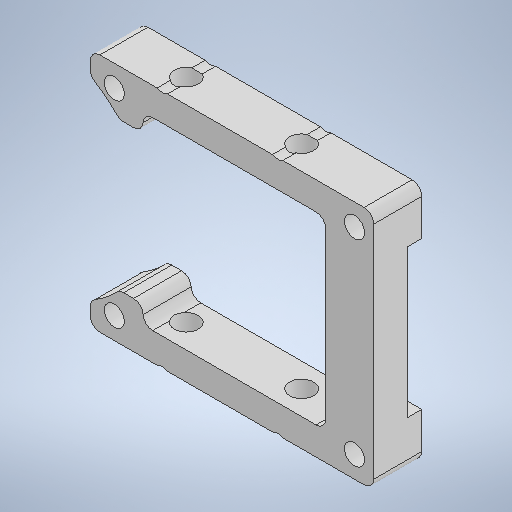
# Autodesk Inventor part: AP3.0_servo-mount
Saved by Autodesk Inventor 2025.1 (Build 291241020, 241B)
## iProperties
Created: 2024-04-22
Part Number: AP3.0_servo-mount
Material: 一般
Document SubType Name: Sheet Metal
Designer: 8326d
Density: 1 g/cm^3
Sheet Metal Rule: Default_mm
Appearance: 既定
Author: 8326d
## iProperties of the stored document T3.0_servo-mount_3D プリント.ipt
Created: 2024-09-23
Part Number: T3.0_servo-mount_3D プリント
Material: 一般
Document SubType Name: Modeling
Designer: 8326d
Density: 1 g/cm^3
Appearance: 既定
Author: 8326d
Autodesk Inventor part; units mm, degrees
ref_plane "YZ Plane" through (0, 0, 0) normal (1, 0, 0) x (0, 1, 0)
ref_plane "XZ Plane" through (0, 0, 0) normal (0, 1, 0) x (-1, 0, 0)
ref_plane "XY Plane" through (0, 0, 0) normal (0, 0, 1) x (1, 0, 0)
sketch "スケッチ1" plane through (0, 0, 0) normal (0, 0, 1) x (1, 0, 0)
  line L0 (-14.75, -12.5) -> (14.75, -12.5)
  line L1 (14.75, -12.5) -> (14.75, 12.5)
  line L2 (14.75, 12.5) -> (-14.75, 12.5)
  line L3 (-14.75, 12.5) -> (-14.75, -12.5)
  line L4 (-14.75, -12.5) -> (14.75, 12.5) construction
  line L5 (14.75, -12.5) -> (-14.75, 12.5) construction
  point P0 (0, 0)
  dimension "d0" = 29.5
  dimension "d1" = 25
  measures "d0" distance of L1.end L2.end
  measures "d1" distance of L0.end L1.end
extrude "プレート1" add sketch "スケッチ1" along normal blind 5
sketch "スケッチ2" plane through (0, 0, 5) normal (0, 0, 1) x (1, 0, 0)
  line L0 (-12.25, -10.25) -> (12.75, -10.25) construction
  line L1 (12.75, -10.25) -> (12.75, 10.25) construction
  line L2 (12.75, 10.25) -> (-12.25, 10.25) construction
  line L3 (-12.25, 10.25) -> (-12.25, -10.25) construction
  line L4 (-12.25, -10.25) -> (12.75, 10.25) construction
  line L5 (12.75, -10.25) -> (-12.25, 10.25) construction
  line L6 (14.75, 12.5) -> (14.75, -12.5) construction
  point P0 (0, 0)
  point P1 (0.25, 0)
  dimension "d3" = 25
  dimension "d4" = 20.5
  dimension "d5" = 2
  constraints: 12 end point, 2 midpoint, 2 parallel, 1 horizontal, 1 horizontal alignment, 1 perpendicular
  measures "d3" distance of L2.end L1.end
  measures "d4" distance of L1.end L0.end
  measures "d5" distance between parallel lines of L6 L1
hole "穴1" at (-12.25, 10.25, 5) at (12.75, 10.25, 5) at (12.75, -10.25, 5) at (-12.25, -10.25, 5) direction (0, 0, -1) diameter 2.1 end through all
sketch "スケッチ3" plane through (0, 0, 0) normal (0, 0, -1) x (-1, 0, 0)
  line L0 (-14.75, -12.5) -> (-14.75, 12.5) projected
  line L1 (14.75, 12.5) -> (14.75, -12.5) projected
  line L2 (-14.75, 7.7) -> (14.75, 7.7)
  line L3 (14.75, -7.7) -> (-14.75, -7.7)
  line L4 (-14.75, 12.5) -> (14.75, 12.5) projected
  line L5 (14.75, -12.5) -> (-14.75, -12.5) projected
  point P0 (0, 0)
  dimension "d13" = 4.8
  dimension "d14" = 4.8
  constraints: 4 end point, 4 point on line, 3 perpendicular
  measures "d13" distance between parallel lines of L4 L2
  measures "d14" distance between parallel lines of L5 L3
extrude "押し出し1" cut sketch "スケッチ3" against normal blind 1.5 contours L0 L2 L1 L3
sketch "スケッチ4" plane through (0, 0, 5) normal (0, 0, 1) x (1, 0, 0)
  line L0 (-14.75, 12.5) -> (14.75, 12.5) projected
  line L1 (14.75, -12.5) -> (-14.75, -12.5) projected
  circle A0 centre (-20.25, 0) radius 11.5
  line L2 (14.75, 12.5) -> (14.75, -12.5) projected
  line L3 (9.75, -9.6) -> (-9.25, -9.6)
  line L4 (-9.25, -9.6) -> (-9.25, 9.6)
  line L5 (-9.25, 9.6) -> (9.75, 9.6)
  line L6 (9.75, 9.6) -> (9.75, -9.6)
  line L7 (9.75, -9.6) -> (-9.25, 9.6) construction
  line L8 (-9.25, -9.6) -> (9.75, 9.6) construction
  line L9 (-9.25, 7.7) -> (-11.7083, 7.7)
  line L10 (-11.7083, 7.7) -> (-11.7083, -7.7)
  line L11 (-11.7083, -7.7) -> (-9.25, -7.7)
  line L12 (-9.25, -7.7) -> (-9.25, 7.7)
  line L13 (14.75, 7.7) -> (-14.75, 7.7) projected
  point P0 (0, 0)
  point P1 (14.75, 0)
  point P2 (0.25, 0)
  point P3 (-9.25, 0)
  point P4 (-11.7083, 7.7)
  dimension "d18" = 23
  dimension "d17" = 35
  dimension "d19" = 5
  dimension "d20" = 2.9
  dimension "d22" = 19
  constraints: 20 end point, 4 midpoint, 4 parallel, 3 horizontal alignment, 2 horizontal, 2 perpendicular, 1 collinear, 1 point on line, 3 other
  measures "d17" distance from line of L2 point (-20.25, 0)
  measures "d19" distance between parallel lines of L2 L6
  measures "d20" distance between parallel lines of L0 L5
  measures "d22" distance between parallel lines of L6 L12
extrude "押し出し2" cut sketch "スケッチ4" against normal through all
fillet "フィレット1" radius 1 14 edges at (-9.25, 9.6, 2.5) (-9.25, -9.6, 2.5) (9.75, -9.6, 2.5) (9.75, 9.6, 2.5) (-9.25, 7.7, 2.5) (-9.25, -7.7, 2.5) (-11.7083, -7.7, 2.5) (-11.7083, 7.7, 2.5) (-14.75, 10.0995, 2.5) (-14.75, -10.0995, 2.5) (-14.75, -12.5, 2.5) (14.75, -12.5, 2.5) (14.75, 12.5, 2.5) (-14.75, 12.5, 2.5)
sketch "スケッチ5" plane through (0, 0, 5) normal (0, 0, 1) x (1, 0, 0)
  line L0 (-13.75, 12.5) -> (13.75, 12.5) projected
  circle A0 centre (-7.25, 13.4) radius 1.05
  circle A1 centre (4.75, 13.4) radius 1.05
  line L1 (14.75, 11.5) -> (14.75, -11.5) projected
  point P0 (0, 0)
  dimension "d26" = 2.1
  dimension "d27" = 2.1
  dimension "d28" = 0.9
  dimension "d29" = 0.9
  dimension "d30" = 12
  dimension "d31" = 10
  constraints: 2 centre point
  measures "d26" diameter of A0
  measures "d27" diameter of A1
  measures "d28" distance from line of L0 A0.centre
  measures "d29" distance from line of L0 A1.centre
  measures "d30" distance of A1.centre A0.centre
  measures "d31" distance from line of L1 A1.centre
extrude "押し出し3" cut sketch "スケッチ5" against normal through all
sketch "スケッチ6" plane through (-6.7092, 12.5, 0) normal (0, 1, 0) x (1, 0, 0)
  line L0 (-1.0817, -5) -> (-1.0817, 0) projected
  line L1 (0, -5) -> (-1.0817, -5) projected
  line L2 (0, 0) -> (0, -5) projected
  line L3 (-1.0817, 0) -> (0, 0) projected
  line L4 (10.9183, -5) -> (10.9183, 0) projected
  line L5 (12, -5) -> (10.9183, -5) projected
  line L6 (12, 0) -> (12, -5) projected
  line L7 (10.9183, 0) -> (12, 0) projected
  line L8 (-1.5408, -5) -> (-1.5408, 0) construction
  line L9 (-1.5408, 0) -> (-1.5408, -5) construction
  line L10 (-1.0817, -2.5) -> (0, -2.5) construction
  line L11 (10.9183, -2.5) -> (12, -2.5) construction
  line L12 (11.4592, -5) -> (11.4592, 0) construction
  point P0 (6.7092, 0)
  point P1 (-0.5408, -2.5)
  point P2 (11.4592, -2.5)
  constraints: 8 end point, 8 midpoint, 1 point on line, 1 vertical
hole "穴2" at (-7.25, 12.5, 2.5) at (4.75, 12.5, 2.5) direction (0, -1, 0) diameter 2.5 end through all
mirror "ミラー1" about plane through (0, 0, 0) normal (0, 1, 0) of "穴2", "押し出し3"
equation "\"d11\" = Thickness"
equation "\"d14\" = d13"
equation "\"d29\" = d28"
equation "\"d2\" = Thickness"
equation "\"BendRadius\" = Thickness"
equation "\"BendReliefWidth\" = Thickness"
equation "\"BendReliefDepth\" = 0.5 * Thickness"
equation "\"TransitionRadius\" = BendRadius"
equation "\"JacobiRadiusSize\" = BendRadius"
equation "\"GapSize\" = Thickness"
equation "\"Thickness\" = 5"
